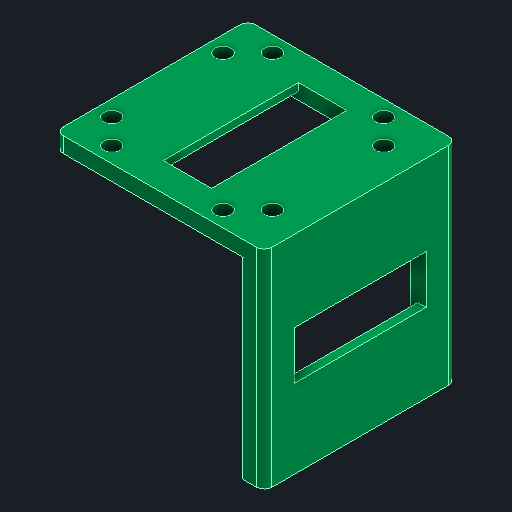
# Autodesk Inventor part: Lens Light Cover
Saved by Autodesk Inventor 2023.4 (Build 274418000, 418)
## iProperties
Created: 2024-07-23
Part Number: Lens Light Cover
Material: Generic
Document SubType Name: Modeling
Designer: xSibe
Density: 1 g/cm^3
Appearance: Plastic Dark Green
Author: xSibe
Autodesk Inventor part; units mm, degrees
ref_plane "YZ Plane" through (0, 0, 0) normal (1, 0, 0) x (0, 1, 0)
ref_plane "XZ Plane" through (0, 0, 0) normal (0, 1, 0) x (-1, 0, 0)
sketch "Sketch1" plane through (0, 0, 0) normal (0, 1, 0) x (-1, 0, 0)
  line L0 (-155.225, -15) -> (-155.225, 15) projected
  line L1 (-155.225, 15) -> (-147.725, 15) projected
  line L2 (-147.725, 15) -> (-147.725, -15) projected
  line L3 (-147.725, -15) -> (-155.225, -15) projected
  circle A0 centre (-171.5, -21.9) radius 1.875 projected
  circle A1 centre (-127.7, 21.9) radius 1.875 projected
  circle A2 centre (-127.7, -21.9) radius 1.875 projected
  circle A3 centre (-171.5, 21.9) radius 1.875 projected
  circle A4 centre (-135.2, 20.8) radius 2.0734 projected
  circle A5 centre (-164, -20.8) radius 2.0734 projected
  circle A6 centre (-135.2, -20.8) radius 2.0734 projected
  circle A7 centre (-128.8, -14.4) radius 2.0734 projected
  circle A8 centre (-128.8, 14.4) radius 2.0734 projected
  circle A9 centre (-164, 20.8) radius 2.0734 projected
  circle A10 centre (-170.4, -14.4) radius 2.0734 projected
  circle A11 centre (-170.4, 14.4) radius 2.0734 projected
  line L4 (-172.5, 24.875) -> (-126.7, 24.875) projected
  arc A12 (-172.5, 24.875) -> (-174.475, 22.9) centre (-172.5, 22.9) ccw projected
  line L5 (-174.475, -22.9) -> (-174.475, 22.9) projected
  arc A13 (-174.475, -22.9) -> (-172.5, -24.875) centre (-172.5, -22.9) ccw projected
  line L6 (-126.7, -24.875) -> (-172.5, -24.875) projected
  arc A14 (-126.7, -24.875) -> (-124.725, -22.9) centre (-126.7, -22.9) ccw projected
  line L7 (-124.725, 22.9) -> (-124.725, -22.9) projected
  arc A15 (-124.725, 22.9) -> (-126.7, 24.875) centre (-126.7, 22.9) ccw projected
  point P0 (0, 0)
ref_plane "Work Plane1" through (124.725, 49.8, -24.875) normal (0, 1, 0) x (0, 0, 1)
extrude "Extrusion1" add sketch "Sketch1" along normal blind 4 from surface at 49.8 contours A0 | A1 | A2 | A3 | L4 A15 L7 A14 L6 A13 L5 A12
sketch "Sketch2" plane through (126.7, 53.8, -24.875) normal (0, 1, 0) x (1, 0, 0)
  line L0 (28.525, -9.875) -> (21.025, -9.875) projected
  line L1 (28.525, -39.875) -> (28.525, -9.875) projected
  line L2 (21.025, -39.875) -> (28.525, -39.875) projected
  line L3 (21.025, -9.875) -> (21.025, -39.875) projected
  circle A0 centre (8.5, -45.675) radius 2.0734 projected
  circle A1 centre (37.3, -4.075) radius 2.0734 projected
  circle A2 centre (8.5, -4.075) radius 2.0734 projected
  circle A3 centre (2.1, -10.475) radius 2.0734 projected
  circle A4 centre (2.1, -39.275) radius 2.0734 projected
  circle A5 centre (37.3, -45.675) radius 2.0734 projected
  circle A6 centre (43.7, -10.475) radius 2.0734 projected
  circle A7 centre (43.7, -39.275) radius 2.0734 projected
  arc A8 (47.775, -1.975) -> (45.8, 0) centre (45.8, -1.975) ccw projected
  line L4 (0, 0) -> (45.8, 0) projected
  arc A9 (0, 0) -> (-1.975, -1.975) centre (0, -1.975) ccw projected
  line L5 (-1.975, -47.775) -> (-1.975, -1.975) projected
  arc A10 (-1.975, -47.775) -> (0, -49.75) centre (0, -47.775) ccw projected
  line L6 (45.8, -49.75) -> (0, -49.75) projected
  arc A11 (45.8, -49.75) -> (47.775, -47.775) centre (45.8, -47.775) ccw projected
  line L7 (47.775, -1.975) -> (47.775, -47.775) projected
  line L8 (18.525, -42.375) -> (31.025, -42.375)
  line L9 (31.025, -42.375) -> (31.025, -7.375)
  line L10 (31.025, -7.375) -> (18.525, -7.375)
  line L11 (18.525, -7.375) -> (18.525, -42.375)
  line L12 (45.8, 0) -> (52.05, 0)
  line L13 (52.05, 0) -> (52.05, -49.75)
  line L14 (52.05, -49.75) -> (45.8, -49.75)
  line L15 (45.8, -49.75) -> (45.8, 0)
  line L16 (52.05, -49.75) -> (47.925, -49.75)
  line L17 (47.925, -49.75) -> (47.925, 0)
  line L18 (47.925, 0) -> (52.05, 0)
  line L19 (52.05, 0) -> (52.05, -49.75)
  arc A12 (45.8, -49.875) -> (47.9, -47.775) centre (45.8, -47.775) ccw
  line L20 (45.8, -49.875) -> (0, -49.875)
  arc A13 (-2.1, -47.775) -> (0, -49.875) centre (0, -47.775) ccw
  line L21 (-2.1, -47.775) -> (-2.1, -1.975)
  arc A14 (0, 0.125) -> (-2.1, -1.975) centre (0, -1.975) ccw
  line L22 (0, 0.125) -> (45.8, 0.125)
  arc A15 (47.9, -1.975) -> (45.8, 0.125) centre (45.8, -1.975) ccw
  line L23 (47.9, -1.975) -> (47.9, -47.775)
  line L24 (18.525, -42.375) -> (11.025, -42.375)
  line L25 (11.025, -42.375) -> (11.025, -7.375)
  line L26 (11.025, -7.375) -> (18.525, -7.375)
  line L27 (18.525, -7.375) -> (18.525, -42.375)
  line L28 (31.025, -42.375) -> (38.525, -42.375)
  line L29 (38.525, -42.375) -> (38.525, -7.375)
  line L30 (38.525, -7.375) -> (31.025, -7.375)
  line L31 (31.025, -7.375) -> (31.025, -42.375)
  point P0 (-126.7, -24.875)
  point P1 (46.5137, -49.75)
  point P2 (46.5137, 0)
  point P3 (31.025, -7.375)
  point P4 (18.525, -7.375)
  dimension "d2" = 2.5
  dimension "d3" = 6.25
  dimension "d4" = 4.125
  dimension "d15" = 0.125
  dimension "d16" = 7.5
  dimension "d17" = 7.5
  constraints: 48 end point, 8 parallel, 8 point on circle, 4 centre point, 4 horizontal, 4 perpendicular, 2 collinear, 1 point on line, 10 other
  measures "d2" distance between parallel lines of L3 L11
  measures "d3" distance of L6.start L13.end
  measures "d4" distance of L17.end L18.end
  measures "d15" radial gap between concentric circles of A11 A12
  measures "d16" distance of L25.end L26.end
  measures "d17" distance of L30.end L29.end
extrude "Extrusion2" cut sketch "Sketch2" against normal up to surface (4 mm away) contours L11 L10 L9 L8
extrude "Extrusion3" add sketch "Sketch2" against normal up to surface (4 mm away) contours A8 L12 A15 L23 A12 L14 A11 L7 | L12 L17 L14 A12 L23 A15 | L12 L13 L14 L17
extrude "Extrusion4" add sketch "Sketch2" against normal blind 49.8 from surface at -4 contours L12 L17 L14 A12 L23 A15 | L12 L13 L14 L17
extrude "Extrusion5" cut sketch "Sketch2" along normal blind 2 from surface at -4 contours L24 L25 L26 L11 | L9 L30 L29 L28
fillet "Fillet1" radius 2 2 edges at (178.75, 26.9, 24.875) (178.75, 26.9, -24.875)
sketch "Sketch3" plane through (178.75, 53.8, 22.875) normal (1, 0, 0) x (0, 0, -1)
  line L0 (7.875, -23.425) -> (7.875, -30.925) projected
  line L1 (7.875, -30.925) -> (37.875, -30.925) projected
  line L2 (37.875, -30.925) -> (37.875, -23.425) projected
  line L3 (37.875, -23.425) -> (7.875, -23.425) projected
  line L4 (5.825, -11.7) -> (39.925, -11.7) projected
  line L5 (39.925, -46.1) -> (39.925, -11.7) projected
  line L6 (5.825, -46.1) -> (39.925, -46.1) projected
  line L7 (5.825, -11.7) -> (5.825, -46.1) projected
  line L8 (5.375, -20.925) -> (5.375, -33.425)
  line L9 (5.375, -33.425) -> (40.375, -33.425)
  line L10 (40.375, -33.425) -> (40.375, -20.925)
  line L11 (40.375, -20.925) -> (5.375, -20.925)
  point P0 (22.875, -53.8)
  point P1 (39.925, -20.925)
  point P2 (5.825, -20.925)
  point P3 (5.825, -33.425)
  point P4 (39.925, -33.425)
  dimension "d12" = 2.5
  constraints: 8 end point, 3 other
  measures "d12" distance between parallel lines of L3 L11
extrude "Extrusion6" cut sketch "Sketch3" against normal up to surface (4.15 mm away) contours L3 L2 L1 L0 | L11 L5 L9 L7
sketch "Sketch4" plane through (178.75, 53.8, 22.875) normal (1, 0, 0) x (0, 0, -1)
  line L0 (5.825, -20.925) -> (39.925, -20.925) projected
  line L1 (39.925, -20.925) -> (39.925, -33.425) projected
  line L2 (39.925, -33.425) -> (5.825, -33.425) projected
  line L3 (5.825, -33.425) -> (5.825, -20.925) projected
  line L4 (45.75, 0) -> (45.75, -53.8) projected
  line L5 (0, 0) -> (45.75, 0) projected
  line L6 (0, -53.8) -> (0, 0) projected
  line L7 (45.75, -53.8) -> (0, -53.8) projected
  line L8 (5.825, -20.925) -> (39.925, -20.925)
  line L9 (39.925, -20.925) -> (39.925, -13.425)
  line L10 (39.925, -13.425) -> (5.825, -13.425)
  line L11 (5.825, -13.425) -> (5.825, -20.925)
  line L12 (5.825, -33.425) -> (39.925, -33.425)
  line L13 (39.925, -33.425) -> (39.925, -40.925)
  line L14 (39.925, -40.925) -> (5.825, -40.925)
  line L15 (5.825, -40.925) -> (5.825, -33.425)
  point P0 (22.875, -53.8)
  point P1 (39.925, -20.925)
  dimension "d20" = 7.5
  dimension "d21" = 7.5
  constraints: 16 end point, 4 parallel, 2 horizontal, 2 perpendicular, 1 collinear, 1 point on line
  measures "d20" distance of L9.end L8.end
  measures "d21" distance of L12.end L13.end
extrude "Extrusion7" cut sketch "Sketch4" along normal blind 2 from surface at -4.15 contours L11 L10 L9 L0 | L2 L13 L14 L15
chamfer "Chamfer1" distance 2 angle 45 2 edges at (174.6, 40.375, 0) (174.6, 12.875, 0)
body "Solid1"
